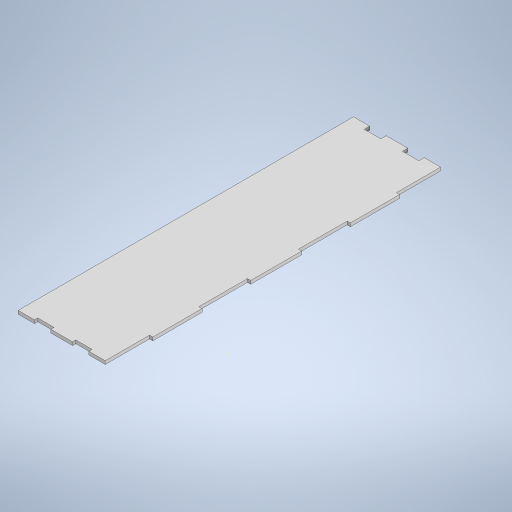
# Autodesk Inventor part: mieng_ben_3mm
Saved by Autodesk Inventor 2023 (Build 270158000, 158)
## iProperties
Created: 2022-11-20
Part Number: mieng_ben_3mm
Material: Generic
Document SubType Name: Modeling
Designer: ADMIN
Density: 1 g/cm^3
Appearance: Default
Author: ADMIN
Autodesk Inventor part; units mm, degrees
ref_plane "YZ Plane" through (0, 0, 0) normal (1, 0, 0) x (0, 1, 0)
ref_plane "XZ Plane" through (0, 0, 0) normal (0, 1, 0) x (-1, 0, 0)
ref_plane "XY Plane" through (0, 0, 0) normal (0, 0, 1) x (1, 0, 0)
sketch "Sketch1" plane through (0, 0, 0) normal (0, 1, 0) x (-1, 0, 0)
  point P0 (0, 0)
sketch "Sketch2" plane through (0, 0, 0) normal (0, 1, 0) x (-1, 0, 0)
  line L0 (128.8824, 62.1664) -> (128.8824, -237.8336)
  line L1 (48.8824, 24.5697) -> (45.8824, 24.5697)
  line L2 (48.8824, -65.4156) -> (45.8824, -65.4156)
  line L3 (48.8824, -20.7764) -> (45.8824, -20.7764)
  line L4 (48.8824, -202.2369) -> (45.8824, -202.2369)
  line L5 (48.8824, -156.8908) -> (45.8824, -156.8908)
  line L6 (48.8824, -112.2516) -> (45.8824, -112.2516)
  line L7 (48.8824, 24.5697) -> (48.8824, 62.1664)
  line L8 (48.8824, 24.5697) -> (48.8824, 65.1664)
  line L9 (48.8824, -65.4156) -> (48.8824, -20.7764)
  line L10 (48.8824, -65.4156) -> (48.8824, -20.7764)
  line L11 (48.8824, -237.8336) -> (48.8824, -202.2369)
  line L12 (48.8824, -156.8908) -> (48.8824, -112.2516)
  line L13 (48.8824, -156.8908) -> (48.8824, -112.2516)
  line L14 (45.8824, -20.7764) -> (45.8824, 24.5697)
  line L15 (45.8824, -202.2369) -> (45.8824, -156.8908)
  line L16 (45.8824, -112.2516) -> (45.8824, -65.4156)
  line L17 (128.8824, -242.8336) -> (128.8824, -237.8336)
  line L18 (48.8824, -242.8336) -> (63.8824, -242.8336)
  line L19 (63.8824, -242.8336) -> (63.8824, -237.8336)
  line L20 (63.8824, -237.8336) -> (78.8824, -237.8336)
  line L21 (78.8824, -237.8336) -> (78.8824, -242.8336)
  line L22 (98.8824, -237.8336) -> (98.8824, -242.8336)
  line L23 (113.8824, -242.8336) -> (113.8824, -237.8336)
  line L24 (128.8824, -242.8336) -> (113.8824, -242.8336)
  line L25 (113.8824, -237.8336) -> (98.8824, -237.8336)
  line L26 (78.8824, -237.8336) -> (63.8824, -237.8336)
  line L27 (98.8824, -242.8336) -> (78.8824, -242.8336)
  line L28 (113.8824, 65.1664) -> (113.8824, 62.1664)
  line L29 (98.8824, 62.1664) -> (98.8824, 65.1664)
  line L30 (78.8824, 62.1664) -> (78.8824, 65.1664)
  line L31 (63.8824, 65.1664) -> (63.8824, 62.1664)
  line L32 (128.8824, 62.1664) -> (128.8824, 65.1664)
  line L33 (48.8824, 65.1664) -> (63.8824, 65.1664)
  line L34 (63.8824, 62.1664) -> (78.8824, 62.1664)
  line L35 (98.8824, 62.1664) -> (113.8824, 62.1664)
  line L36 (78.8824, 65.1664) -> (98.8824, 65.1664)
  line L37 (113.8824, 65.1664) -> (128.8824, 65.1664)
  line L38 (63.8824, -237.8336) -> (75.0605, -237.8336)
  line L39 (48.8824, -242.8336) -> (48.8824, -237.8336)
  point P0 (0, 0)
  point P1 (106.3824, -237.8336)
  point P2 (106.3824, 62.1664)
  point P3 (121.3824, 65.1664)
  point P4 (47.3824, -202.2369)
  dimension "d0" = 80
  dimension "d1" = 15
  dimension "d2" = 15
  dimension "d3" = 300
  dimension "d4" = 80
  dimension "d5" = 3
  dimension "d6" = 5
  dimension "d7" = 44.6392
  dimension "d8" = 37.5967
  dimension "d9" = 44.6392
  dimension "d10" = 40.5967
  dimension "d11" = 45.3461
  dimension "d12" = 46.8359
  dimension "d13" = 45.3461
  dimension "d14" = 20
  dimension "d15" = 15
  dimension "d16" = 15
  dimension "d17" = 15
  dimension "d18" = 15
  dimension "d19" = 15
  dimension "d20" = 15
  dimension "d21" = 20
  dimension "d22" = 308
  constraints: 80 end point, 16 perpendicular, 8 parallel, 5 horizontal, 4 midpoint, 2 vertical, 1 point on line
  measures "d0" distance of L17.end L11.start
  measures "d1" distance of L18.start L19.start
  measures "d2" distance of L21.start L19.end
  measures "d3" distance of point (106.382, -237.834) point (106.382, 62.166)
  measures "d4" distance between parallel lines of L8 L0
  measures "d5" vertical distance of L28.end point (121.382, 65.166)
  measures "d6" distance between parallel lines of L25 L24
  measures "d7" distance of L9.start L9.end
  measures "d8" distance of L1.start L7.end
  measures "d9" distance of L5.start L6.start
  measures "d10" distance from line of L18 point (47.382, -202.237)
  measures "d11" distance of L4.end L5.end
  measures "d12" distance of L16.start L2.end
  measures "d13" distance of L3.end L14.end
  measures "d14" distance of L36.start L29.end
  measures "d15" distance of L29.start L28.end
  measures "d16" distance of L28.start L37.end
  measures "d17" distance of L33.start L31.start
  measures "d18" distance of L34.start L30.start
  measures "d19" distance of L24.start L24.end
  measures "d20" distance of L25.start L22.start
  measures "d21" distance of L27.start L27.end
  measures "d22" distance between parallel lines of L24 L37
extrude "Extrusion1" add sketch "Sketch2" along normal blind 3
body "Solid1"
